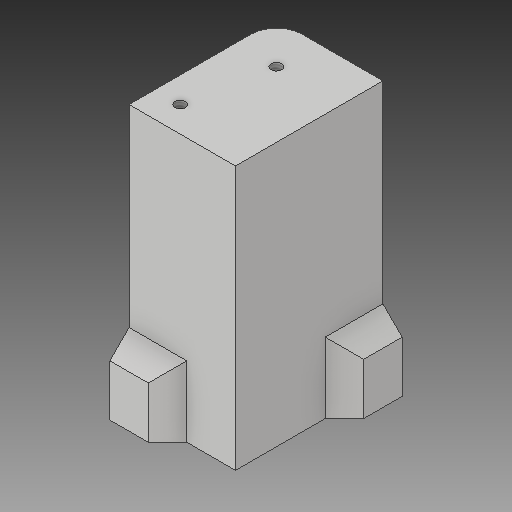
# Autodesk Inventor part: WheelIntakeBrace
Saved by Autodesk Inventor 2017 (Build 210142000, 142)
## iProperties
Created: 2017-12-16
Part Number: WheelIntakeBrace
Material: Generic
Document SubType Name: Modeling
Designer: User
Density: 1 g/cm^3
Appearance: Default
Mass: 22.8813 g
Surface Area: 106.595 cm^2
Volume: 22.8813 cm^3
Author: User
Autodesk Inventor part; units mm, degrees
ref_plane "YZ Plane" through (0, 0, 0) normal (1, 0, 0) x (0, 1, 0)
ref_plane "XZ Plane" through (0, 0, 0) normal (0, 1, 0) x (-1, 0, 0)
ref_plane "XY Plane" through (0, 0, 0) normal (0, 0, 1) x (1, 0, 0)
sketch "Sketch1" plane through (0, 0, 0) normal (1, 0, 0) x (0, 1, 0)
  line L0 (0, 0) -> (65.278, 0)
  line L1 (65.278, 0) -> (65.278, -16.1544)
  line L2 (0, -16.1544) -> (0, 0)
  line L3 (0, 0) -> (0, -20.066)
  line L4 (65.278, 0) -> (0, 0)
  line L5 (0, 0) -> (0, -36.5125)
  line L6 (0, -36.5125) -> (65.278, -36.5125)
  line L7 (65.278, -36.5125) -> (65.278, 0)
  dimension "d0" = 65.278
  dimension "d1" = 16.1544
  dimension "d11" = 36.5125
  constraints: 16 end point, 3 parallel, 2 horizontal, 2 perpendicular, 1 point on line
  measures "d0" distance of L1.end L2.start
  measures "d1" distance of L0.end L1.end
  measures "d11" distance of L5.end L4.end
extrude "Extrusion1" add sketch "Sketch1" along normal blind 4.7625
sketch "Sketch3" plane through (0, 0, 0) normal (0, 0, 1) x (1, 0, 0)
  line L0 (0, 65.278) -> (0, 0) projected
  line L1 (0, 0) -> (4.7625, 0) projected
  line L2 (4.7625, 65.278) -> (4.7625, 0) projected
  line L3 (0, 65.278) -> (4.7625, 65.278) projected
  line L4 (4.7625, 65.278) -> (4.7625, 0) projected
  line L5 (4.7625, 65.278) -> (-21.59, 65.278)
  line L6 (-21.59, 65.278) -> (-21.59, 0)
  line L7 (-21.59, 0) -> (4.7625, 0)
  line L8 (4.7625, 0) -> (4.7625, 65.278)
  dimension "d12" = 26.3525
  constraints: 8 end point, 2 parallel, 1 horizontal, 1 perpendicular
  measures "d12" distance of L7.end L6.end
extrude "Extrusion3" add sketch "Sketch3" against normal blind 4.7625 contours L0 L7 L6 L5
sketch "Sketch4" plane through (0, 65.278, -36.5125) normal (0, 1, 0) x (1, 0, 0)
  line L0 (0, 0) -> (0, -31.75) projected
  line L1 (-21.59, -31.75) -> (0, -31.75) projected
  line L2 (-21.59, -36.5125) -> (-21.59, -31.75) projected
  line L3 (4.7625, -36.5125) -> (-21.59, -36.5125) projected
  line L4 (4.7625, 0) -> (4.7625, -36.5125) projected
  line L5 (0, 0) -> (4.7625, 0) projected
  line L6 (-21.59, -31.75) -> (0, -31.75) projected
  line L7 (-21.59, -31.75) -> (-21.59, 0)
  line L8 (0, 0) -> (-21.59, 0)
  line L9 (-21.59, 0) -> (0, 0)
  line L10 (0, 0) -> (0, -31.75)
  line L11 (0, -31.75) -> (-21.59, -31.75)
  line L12 (-21.59, -31.75) -> (-21.59, 0)
  point P0 (0, -36.5125)
  dimension "d15" = 31.75
  dimension "d16" = 21.59
  dimension "d50" = 31.75
  dimension "d51" = 21.59
  constraints: 12 end point, 2 horizontal, 2 parallel, 1 perpendicular, 1 vertical
  measures "d15" distance of L1.start L7.end
  measures "d16" distance of L0.start L8.end
  measures "d50" distance of L0.start L0.end
  measures "d51" distance of L1.start L0.end
extrude "Extrusion4" add sketch "Sketch4" against normal blind 4.7625
fillet "Fillet1" radius 1.5875 3 edges at (0, 60.5155, -20.6375) (-10.795, 60.5155, -4.7625) (0, 30.2578, -4.7625)
sketch "Sketch6" plane through (0, 0, -36.5125) normal (0, -1, 0) x (1, 0, 0)
  line L0 (0, 30.1625) -> (0, 0) projected
  line L1 (0, 0) -> (4.7625, 0) projected
  line L2 (4.7625, 36.5125) -> (4.7625, 0) projected
  line L3 (-21.59, 36.5125) -> (4.7625, 36.5125) projected
  line L4 (-21.59, 36.5125) -> (-21.59, 31.75) projected
  line L5 (-1.5875, 31.75) -> (-21.59, 31.75) projected
  arc A0 (0, 30.1625) -> (-1.5875, 31.75) centre (-1.5875, 30.1625) ccw projected
  line L6 (0, 0) -> (9.525, 0)
  line L7 (9.525, 0) -> (9.525, 9.525)
  line L8 (9.525, 9.525) -> (0, 9.525)
  line L9 (0, 9.525) -> (0, 0)
  line L10 (-21.59, 36.5125) -> (-21.59, 31.75) projected
  line L11 (-21.59, 31.75) -> (-12.065, 31.75)
  line L12 (-12.065, 31.75) -> (-12.065, 41.275)
  line L13 (-12.065, 41.275) -> (-21.59, 41.275)
  line L14 (-21.59, 41.275) -> (-21.59, 31.75)
  point P0 (0, 36.5125)
  dimension "d24" = 9.525
  dimension "d25" = 9.525
  dimension "d26" = 9.525
  dimension "d27" = 9.525
  constraints: 16 end point, 4 parallel, 2 horizontal, 2 perpendicular
  measures "d24" distance of L8.end L7.end
  measures "d25" distance of L7.end L6.end
  measures "d26" distance of L13.end L12.end
  measures "d27" distance of L12.end L11.end
extrude "Extrusion5" add sketch "Sketch6" against normal blind 12.7 contours L8 L2 L1 L0 | L8 L7 L6 L2 | L5 L4 L3 L12 | L3 L14 L13 L12
chamfer "Chamfer1" distance 4.7625 angle 45 4 edges at (4.7625, 6.35, -26.9875) (-12.065, 6.35, 0) (4.7625, 12.7, -31.75) (-16.8275, 12.7, 0)
sketch "Sketch8" plane through (-21.59, 0, -4.7625) normal (0, -1, 0) x (1, 0, 0)
  line L0 (20.0025, 0) -> (0, 0) projected
  arc A0 (21.59, -1.5875) -> (20.0025, 0) centre (20.0025, -1.5875) ccw projected
  line L1 (21.59, -1.5875) -> (21.59, -31.75) projected
  line L2 (21.59, -31.75) -> (31.115, -31.75) projected
  line L3 (31.115, -31.75) -> (31.115, -22.225) projected
  line L4 (26.3525, -17.4625) -> (31.115, -22.225) projected
  line L5 (26.3525, 4.7625) -> (26.3525, -17.4625) projected
  line L6 (14.2875, 4.7625) -> (26.3525, 4.7625) projected
  line L7 (9.525, 9.525) -> (14.2875, 4.7625) projected
  line L8 (9.525, 9.525) -> (0, 9.525) projected
  line L9 (0, 9.525) -> (0, 0) projected
  line L10 (26.3525, 4.7625) -> (0, 4.7625) projected
  point P0 (21.59, 4.7625)
  point P1 (4.7625, 4.7625)
  point P2 (26.3525, -26.9875)
  constraints: 1 point on line
hole "Hole1" at (-16.8275, 0, 0) at (4.7625, 0, -31.75) direction (0, 1, 0) diameter 2.6416 depth 12.7 tip angle 118 thread size "6-32 UNC" class "2B" standard "ANSI Unified Screw Threads"
sketch "Sketch9" plane through (4.7625, 65.278, 0) normal (0, 1, 0) x (1, 0, 0)
  line L0 (-26.3525, 36.5125) -> (0, 36.5125) projected
  line L1 (-26.3525, 0) -> (-26.3525, 36.5125) projected
  line L2 (0, 0) -> (-26.3525, 0) projected
  line L3 (0, 36.5125) -> (0, 0) projected
  point P0 (-4.7625, 0)
  point P1 (-20.0025, 6.35)
  point P2 (-16.1925, 26.3525)
  dimension "d52" = 6.35
  dimension "d56" = 10.16
  dimension "d57" = 6.35
  dimension "d58" = 10.16
  measures "d52" distance from line of L2 point (-20.002, 6.35)
  measures "d56" distance from line of L1 point (-16.192, 26.352)
  measures "d57" distance from line of L1 point (-20.002, 6.35)
  measures "d58" distance from line of L0 point (-16.192, 26.352)
hole "Hole2" at (-15.24, 65.278, -6.35) at (-11.43, 65.278, -26.3525) direction (0, -1, 0) diameter 2.6416 end through all thread size "6-32 UNC" class "2B" standard "ANSI Unified Screw Threads"
fillet "Fillet2" radius 6.35 1 edges at (-21.59, 62.8968, -36.5125)
equation "\"d15\" = d50"
equation "\"d16\" = d51"
body "Solid1"
